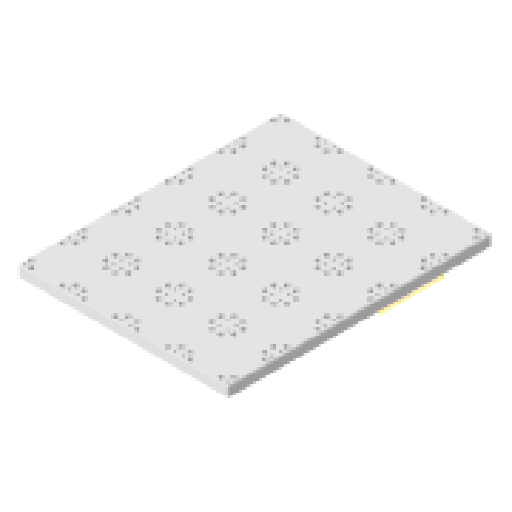
# Autodesk Inventor part: 00_Baseplate_Lightsheet
Saved by Autodesk Inventor 2025.1 (Build 291241020, 241B)
## iProperties
Created: 2024-02-01
Part Number: 00_Baseplate_Lightsheet
Material: Generisch
Document SubType Name: Modeling
Designer: diederichbenedict
Density: 1 g/cm^3
Appearance: Vorgabe
Author: diederichbenedict
Autodesk Inventor part; units mm, degrees
ref_plane "YZ Plane" through (0, 0, 0) normal (1, 0, 0) x (0, 1, 0)
ref_plane "XZ Plane" through (0, 0, 0) normal (0, 1, 0) x (-1, 0, 0)
ref_plane "XY Plane" through (0, 0, 0) normal (0, 0, 1) x (1, 0, 0)
ref_plane "Arbeitsebene1" through (0, 0, 0) normal (0, 0, 1) x (1, 0, 0)
sketch "Skizze1" plane through (0, 0, 0) normal (0, 0, 1) x (1, 0, 0)
  circle A0 centre (27, 33.3) radius 3 construction
  circle A1 centre (-8.3, 27) radius 3 construction
  circle A2 centre (-2, -8.3) radius 3 construction
  circle A3 centre (33.3, -2) radius 3 construction
  circle A4 centre (27, -8.3) radius 3 construction
  circle A5 centre (-8.3, -2) radius 3 construction
  circle A6 centre (-2, 33.3) radius 3 construction
  circle A7 centre (33.3, 27) radius 3 construction
  line L0 (27.5, 29.5) -> (-2.5, 29.5) construction
  arc A8 (29.5, 27.5) -> (27.5, 29.5) centre (27.5, 27.5) ccw construction
  line L1 (29.5, 27.5) -> (29.5, -2.5) construction
  arc A9 (27.5, -4.5) -> (29.5, -2.5) centre (27.5, -2.5) ccw construction
  line L2 (-2.5, -4.5) -> (27.5, -4.5) construction
  arc A10 (-4.5, -2.5) -> (-2.5, -4.5) centre (-2.5, -2.5) ccw construction
  line L3 (-4.5, -2.5) -> (-4.5, 27.5) construction
  arc A11 (-2.5, 29.5) -> (-4.5, 27.5) centre (-2.5, 27.5) ccw construction
  circle A12 centre (33.5, 33.5) radius 2.5 construction
  circle A13 centre (-8.5, -8.5) radius 2.5 construction
  circle A14 centre (33.5, -8.5) radius 2.5 construction
  circle A15 centre (-8.5, 33.5) radius 2.5 construction
  line L4 (-11.75, -10.5) -> (-11.75, 8.25) construction
  arc A16 (-11.75, -10.5) -> (-10.5, -11.75) centre (-10.5, -10.5) ccw construction
  line L5 (8.25, -11.75) -> (-10.5, -11.75) construction
  line L6 (8.25, -13.8774) -> (8.25, -11.75) construction
  arc A17 (7.4056, -14.8652) -> (8.25, -13.8774) centre (7.25, -13.8774) ccw construction
  arc A18 (7.4056, -14.8652) -> (7.6, -17.35) centre (7.6, -16.1) ccw construction
  line L7 (17.4, -17.35) -> (7.6, -17.35) construction
  arc A19 (17.4, -17.35) -> (17.5944, -14.8652) centre (17.4, -16.1) ccw construction
  arc A20 (16.75, -13.8774) -> (17.5944, -14.8652) centre (17.75, -13.8774) ccw construction
  line L8 (16.75, -11.75) -> (16.75, -13.8774) construction
  line L9 (35.5, -11.75) -> (16.75, -11.75) construction
  arc A21 (35.5, -11.75) -> (36.75, -10.5) centre (35.5, -10.5) ccw construction
  line L10 (36.75, 6.4875) -> (36.75, -10.5) construction
  arc A22 (36.75, 6.4875) -> (36.556, 6.5217) centre (36.65, 6.4875) ccw construction
  arc A23 (31.3, 7.45) -> (36.556, 6.5217) centre (34.01, 7.45) ccw construction
  line L11 (31.3, 17.55) -> (31.3, 7.45) construction
  arc A24 (36.556, 18.4783) -> (31.3, 17.55) centre (34.01, 17.55) ccw construction
  arc A25 (36.556, 18.4783) -> (36.75, 18.5125) centre (36.65, 18.5125) ccw construction
  line L12 (36.75, 35.5) -> (36.75, 18.5125) construction
  arc A26 (36.75, 35.5) -> (35.5, 36.75) centre (35.5, 35.5) ccw construction
  line L13 (18.5125, 36.75) -> (35.5, 36.75) construction
  arc A27 (18.5125, 36.75) -> (18.4783, 36.556) centre (18.5125, 36.65) ccw construction
  arc A28 (17.55, 31.3) -> (18.4783, 36.556) centre (17.55, 34.01) ccw construction
  line L14 (7.45, 31.3) -> (17.55, 31.3) construction
  arc A29 (6.5217, 36.556) -> (7.45, 31.3) centre (7.45, 34.01) ccw construction
  arc A30 (6.5217, 36.556) -> (6.4875, 36.75) centre (6.4875, 36.65) ccw construction
  line L15 (-10.5, 36.75) -> (6.4875, 36.75) construction
  arc A31 (-10.5, 36.75) -> (-11.75, 35.5) centre (-10.5, 35.5) ccw construction
  line L16 (-11.75, 16.75) -> (-11.75, 35.5) construction
  line L17 (-13.8774, 16.75) -> (-11.75, 16.75) construction
  arc A32 (-14.8652, 17.5944) -> (-13.8774, 16.75) centre (-13.8774, 17.75) ccw construction
  arc A33 (-14.8652, 17.5944) -> (-17.35, 17.4) centre (-16.1, 17.4) ccw construction
  line L18 (-17.35, 7.6) -> (-17.35, 17.4) construction
  arc A34 (-17.35, 7.6) -> (-14.8652, 7.4056) centre (-16.1, 7.6) ccw construction
  arc A35 (-13.8774, 8.25) -> (-14.8652, 7.4056) centre (-13.8774, 7.25) ccw construction
  line L19 (-11.75, 8.25) -> (-13.8774, 8.25) construction
  line L20 (-12.5, 7.5) -> (-12.5, -10.5) construction
  line L21 (-12.5, 7.5) -> (-12.5, -10.5)
  line L22 (-10.5, -12.5) -> (7.5, -12.5)
  line L23 (7.5, -12.5) -> (7.5, -13.8774)
  arc A36 (7.2889, -14.1243) -> (7.5, -13.8774) centre (7.25, -13.8774) ccw construction
  arc A37 (7.2889, -14.1243) -> (7.6, -18.1) centre (7.6, -16.1) ccw construction
  line L24 (7.6, -18.1) -> (17.4, -18.1) construction
  arc A38 (17.4, -18.1) -> (17.7111, -14.1243) centre (17.4, -16.1) ccw construction
  arc A39 (17.5, -13.8774) -> (17.7111, -14.1243) centre (17.75, -13.8774) ccw construction
  line L25 (17.5, -13.8774) -> (17.5, -12.5)
  line L26 (17.5, -12.5) -> (35.5, -12.5)
  line L27 (37.5, -10.5) -> (37.5, 6.4875) construction
  arc A40 (37.5, 6.4875) -> (35.8514, 6.7786) centre (36.65, 6.4875) ccw
  arc A41 (32.05, 7.45) -> (35.8514, 6.7786) centre (34.01, 7.45) ccw
  line L28 (32.05, 7.45) -> (32.05, 17.55)
  arc A42 (35.8514, 18.2214) -> (32.05, 17.55) centre (34.01, 17.55) ccw
  arc A43 (35.8514, 18.2214) -> (37.5, 18.5125) centre (36.65, 18.5125) ccw
  line L29 (37.5, 18.5125) -> (37.5, 35.5)
  line L30 (35.5, 37.5) -> (18.5125, 37.5)
  arc A44 (18.5125, 37.5) -> (18.2214, 35.8514) centre (18.5125, 36.65) ccw
  arc A45 (17.55, 32.05) -> (18.2214, 35.8514) centre (17.55, 34.01) ccw
  line L31 (17.55, 32.05) -> (7.45, 32.05)
  arc A46 (6.7786, 35.8514) -> (7.45, 32.05) centre (7.45, 34.01) ccw
  arc A47 (6.7786, 35.8514) -> (6.4875, 37.5) centre (6.4875, 36.65) ccw
  line L32 (6.4875, 37.5) -> (-10.5, 37.5)
  line L33 (-12.5, 35.5) -> (-12.5, 17.5)
  line L34 (-12.5, 17.5) -> (-13.8774, 17.5) construction
  arc A48 (-14.1243, 17.7111) -> (-13.8774, 17.5) centre (-13.8774, 17.75) ccw construction
  arc A49 (-14.1243, 17.7111) -> (-18.1, 17.4) centre (-16.1, 17.4) ccw construction
  line L35 (-18.1, 17.4) -> (-18.1, 7.6) construction
  arc A50 (-18.1, 7.6) -> (-14.1243, 7.2889) centre (-16.1, 7.6) ccw construction
  arc A51 (-13.8774, 7.5) -> (-14.1243, 7.2889) centre (-13.8774, 7.25) ccw construction
  line L36 (-13.8774, 7.5) -> (-12.5, 7.5) construction
  line L37 (-3.4722, -5.75) -> (-4.9445, -8.3) projected
  line L38 (27.5, 29.5) -> (-2.5, 29.5) projected
  arc A52 (-2.5, 29.5) -> (-4.5, 27.5) centre (-2.5, 27.5) ccw projected
  line L39 (-4.5, -2.5) -> (-4.5, 27.5) projected
  arc A53 (-4.5, -2.5) -> (-2.5, -4.5) centre (-2.5, -2.5) ccw projected
  line L40 (-2.5, -4.5) -> (27.5, -4.5) projected
  arc A54 (27.5, -4.5) -> (29.5, -2.5) centre (27.5, -2.5) ccw projected
  line L41 (29.5, 27.5) -> (29.5, -2.5) projected
  arc A55 (29.5, 27.5) -> (27.5, 29.5) centre (27.5, 27.5) ccw projected
  line L42 (33.3, 29.9445) -> (30.75, 28.4722) projected
  line L43 (30.75, 28.4722) -> (30.75, 25.5278) projected
  line L44 (30.75, 25.5278) -> (33.3, 24.0555) projected
  line L45 (33.3, 24.0555) -> (35.85, 25.5278) projected
  line L46 (35.85, 25.5278) -> (35.85, 28.4722) projected
  line L47 (35.85, 28.4722) -> (33.3, 29.9445) projected
  line L48 (24.0555, 33.3) -> (25.5278, 30.75) projected
  line L49 (25.5278, 30.75) -> (28.4722, 30.75) projected
  line L50 (28.4722, 30.75) -> (29.9445, 33.3) projected
  line L51 (29.9445, 33.3) -> (28.4722, 35.85) projected
  line L52 (28.4722, 35.85) -> (25.5278, 35.85) projected
  line L53 (25.5278, 35.85) -> (24.0555, 33.3) projected
  line L54 (33.3, -4.9445) -> (30.75, -3.4722) projected
  line L55 (35.85, -3.4722) -> (33.3, -4.9445) projected
  line L56 (35.85, -0.5278) -> (35.85, -3.4722) projected
  line L57 (33.3, 0.9445) -> (35.85, -0.5278) projected
  line L58 (30.75, -0.5278) -> (33.3, 0.9445) projected
  line L59 (30.75, -3.4722) -> (30.75, -0.5278) projected
  line L60 (24.0555, -8.3) -> (25.5278, -5.75) projected
  line L61 (25.5278, -10.85) -> (24.0555, -8.3) projected
  line L62 (28.4722, -10.85) -> (25.5278, -10.85) projected
  line L63 (29.9445, -8.3) -> (28.4722, -10.85) projected
  line L64 (28.4722, -5.75) -> (29.9445, -8.3) projected
  line L65 (25.5278, -5.75) -> (28.4722, -5.75) projected
  line L66 (-8.3, 29.9445) -> (-5.75, 28.4722) projected
  line L67 (-10.85, 28.4722) -> (-8.3, 29.9445) projected
  line L68 (-10.85, 25.5278) -> (-10.85, 28.4722) projected
  line L69 (-8.3, 24.0555) -> (-10.85, 25.5278) projected
  line L70 (-5.75, 25.5278) -> (-8.3, 24.0555) projected
  line L71 (-5.75, 28.4722) -> (-5.75, 25.5278) projected
  line L72 (0.9445, 33.3) -> (-0.5278, 30.75) projected
  line L73 (-0.5278, 35.85) -> (0.9445, 33.3) projected
  line L74 (-3.4722, 35.85) -> (-0.5278, 35.85) projected
  line L75 (-4.9445, 33.3) -> (-3.4722, 35.85) projected
  line L76 (-3.4722, 30.75) -> (-4.9445, 33.3) projected
  line L77 (-0.5278, 30.75) -> (-3.4722, 30.75) projected
  line L78 (0.9445, -8.3) -> (-0.5278, -5.75) projected
  line L79 (-0.5278, -5.75) -> (-3.4722, -5.75) projected
  line L80 (-3.4722, -5.75) -> (-4.9445, -8.3) projected
  line L81 (-4.9445, -8.3) -> (-3.4722, -10.85) projected
  line L82 (-3.4722, -10.85) -> (-0.5278, -10.85) projected
  line L83 (-0.5278, -10.85) -> (0.9445, -8.3) projected
  line L84 (-8.3, -4.9445) -> (-5.75, -3.4722) projected
  line L85 (-5.75, -3.4722) -> (-5.75, -0.5278) projected
  line L86 (-5.75, -0.5278) -> (-8.3, 0.9445) projected
  line L87 (-8.3, 0.9445) -> (-10.85, -0.5278) projected
  line L88 (-10.85, -0.5278) -> (-10.85, -3.4722) projected
  line L89 (-10.85, -3.4722) -> (-8.3, -4.9445) projected
  circle A56 centre (33.5, 33.5) radius 2.5 construction
  circle A57 centre (-8.5, -8.5) radius 2.5 construction
  circle A58 centre (33.5, -8.5) radius 2.5 construction
  circle A59 centre (-8.5, 33.5) radius 2.5 construction
  line L90 (16.75, -11.75) -> (35.5, -11.75) projected
  line L91 (16.75, -13.8774) -> (16.75, -11.75) projected
  arc A60 (16.75, -13.8774) -> (17.5944, -14.8652) centre (17.75, -13.8774) ccw construction
  arc A61 (17.4, -17.35) -> (17.5944, -14.8652) centre (17.4, -16.1) ccw construction
  line L92 (7.6, -17.35) -> (17.4, -17.35) construction
  arc A62 (7.4056, -14.8652) -> (7.6, -17.35) centre (7.6, -16.1) ccw construction
  arc A63 (7.4056, -14.8652) -> (8.25, -13.8774) centre (7.25, -13.8774) ccw construction
  line L93 (8.25, -11.75) -> (8.25, -13.8774) projected
  line L94 (-10.5, -11.75) -> (8.25, -11.75) projected
  arc A64 (-11.75, -10.5) -> (-10.5, -11.75) centre (-10.5, -10.5) ccw projected
  line L95 (-11.75, 8.25) -> (-11.75, -10.5) projected
  line L96 (-13.8774, 8.25) -> (-11.75, 8.25) construction
  arc A65 (-13.8774, 8.25) -> (-14.8652, 7.4056) centre (-13.8774, 7.25) ccw construction
  arc A66 (-17.35, 7.6) -> (-14.8652, 7.4056) centre (-16.1, 7.6) ccw construction
  line L97 (-17.35, 17.4) -> (-17.35, 7.6) construction
  arc A67 (-14.8652, 17.5944) -> (-17.35, 17.4) centre (-16.1, 17.4) ccw construction
  arc A68 (-14.8652, 17.5944) -> (-13.8774, 16.75) centre (-13.8774, 17.75) ccw construction
  line L98 (-11.75, 16.75) -> (-13.8774, 16.75) construction
  line L99 (-11.75, 35.5) -> (-11.75, 16.75) projected
  arc A69 (-10.5, 36.75) -> (-11.75, 35.5) centre (-10.5, 35.5) ccw projected
  line L100 (6.4875, 36.75) -> (-10.5, 36.75) projected
  arc A70 (6.5217, 36.556) -> (6.4875, 36.75) centre (6.4875, 36.65) ccw projected
  arc A71 (6.5217, 36.556) -> (7.45, 31.3) centre (7.45, 34.01) ccw projected
  line L101 (17.55, 31.3) -> (7.45, 31.3) projected
  arc A72 (17.55, 31.3) -> (18.4783, 36.556) centre (17.55, 34.01) ccw projected
  arc A73 (18.5125, 36.75) -> (18.4783, 36.556) centre (18.5125, 36.65) ccw projected
  line L102 (35.5, 36.75) -> (18.5125, 36.75) projected
  arc A74 (36.75, 35.5) -> (35.5, 36.75) centre (35.5, 35.5) ccw projected
  line L103 (36.75, 18.5125) -> (36.75, 35.5) projected
  arc A75 (36.556, 18.4783) -> (36.75, 18.5125) centre (36.65, 18.5125) ccw projected
  arc A76 (36.556, 18.4783) -> (31.3, 17.55) centre (34.01, 17.55) ccw projected
  line L104 (31.3, 7.45) -> (31.3, 17.55) projected
  arc A77 (31.3, 7.45) -> (36.556, 6.5217) centre (34.01, 7.45) ccw projected
  arc A78 (36.75, 6.4875) -> (36.556, 6.5217) centre (36.65, 6.4875) ccw projected
  line L105 (36.75, -10.5) -> (36.75, 6.4875) projected
  arc A79 (35.5, -11.75) -> (36.75, -10.5) centre (35.5, -10.5) ccw projected
  line L106 (33.5, -8.5) -> (33.5, 33.5) construction
  line L107 (33.5, 33.5) -> (-8.5, 33.5) construction
  line L108 (-8.5, 33.5) -> (-8.5, -8.5) construction
  circle A80 centre (-8.5, -8.5) radius 1.4
  circle A81 centre (-8.5, 33.5) radius 1.4
  circle A82 centre (33.5, 33.5) radius 1.4
  circle A83 centre (33.5, -8.5) radius 1.4
  line L109 (37.5, -10.5) -> (37.5, -12.5)
  line L110 (37.5, -12.5) -> (35.4967, -12.5)
  line L111 (-10.5, -12.5) -> (-12.5, -12.5)
  line L112 (-12.5, -12.5) -> (-12.5, -10.5)
  line L113 (-12.5, 35.5) -> (-12.5, 37.5)
  line L114 (-12.5, 37.5) -> (-10.5, 37.5)
  line L115 (37.5, 35.5) -> (37.5, 37.5)
  line L116 (37.5, 37.5) -> (35.5, 37.5)
  circle A84 centre (12.5, 12.5) radius 25 construction
  line L117 (-8.5, 33.5) -> (33.5, 33.5) construction
  line L118 (33.5, 33.5) -> (33.5, -8.5) construction
  line L119 (33.5, -8.5) -> (-8.5, -8.5) construction
  line L120 (-8.5, -8.5) -> (-8.5, 33.5) construction
  line L121 (-8.5, 33.5) -> (33.5, -8.5) construction
  line L122 (33.5, 33.5) -> (-8.5, -8.5) construction
  line L123 (37.5, -10.5) -> (37.5, 18.5125)
  arc A85 (18.5125, -12.5) -> (18.2214, -14.1486) centre (18.5125, -13.35) ccw
  arc A86 (17.55, -17.95) -> (18.2214, -14.1486) centre (17.55, -15.99) ccw construction
  line L124 (17.55, -17.95) -> (7.45, -17.95) construction
  arc A87 (6.7786, -14.1486) -> (7.45, -17.95) centre (7.45, -15.99) ccw construction
  arc A88 (6.7786, -14.1486) -> (6.4875, -12.5) centre (6.4875, -13.35) ccw
  line L125 (37.5, 37.5) -> (-12.5, 37.5)
  line L126 (-12.5, 37.5) -> (-12.5, -12.5)
  line L127 (-12.5, -12.5) -> (37.5, -12.5)
  line L128 (37.5, -12.5) -> (37.5, 37.5)
  point P0 (0, 0)
  point P1 (6.4875, -12.5)
  point P2 (6.0394, -17.3508)
  point P3 (18.9606, -17.3508)
  point P4 (18.5125, -12.5)
  point P5 (37.5, 6.4875)
  point P6 (18.5125, 37.5)
  point P7 (6.4875, 37.5)
  point P8 (-12.5, 17.5)
  point P9 (-10.4995, -12.5)
  dimension "d17" = 2.8
  dimension "d18" = 2.8
  dimension "d19" = 2.8
  dimension "d20" = 2.8
  dimension "d53" = 42
  dimension "d54" = 42
  constraints: 78 end point, 40 point on circle, 25 centre point, 5 collinear, 5 parallel, 4 coincident, 4 perpendicular, 3 horizontal, 3 tangent, 2 midpoint, 1 point on line, 1 vertical, 27 other
  measures "d17" diameter of A80
  measures "d18" diameter of A81
  measures "d19" diameter of A82
  measures "d20" diameter of A83
  measures "d53" distance of L106.start L119.end
  measures "d54" distance of L117.end L106.start
extrude "Extrusion1" add sketch "Skizze1" along normal blind 10.5 contours L126 L33 L113 L114 L32 A47 A46 L31 A45 A44 L30 L116 L115 L29 A43 A42 L28 A41 A40 L123 L109 L110 L26 L127 L22 L111 L112 L21 | L125 A44 A45 L31 A46 A47 | L123 A40 A41 L28 A42 A43 | A55 L41 A54 L40 A53 L39 A52 L38
sketch "Skizze3" plane through (0, 0, 10.5) normal (0, 0, 1) x (1, 0, 0)
  circle A0 centre (33.5, -8.5) radius 1.4 projected
  circle A1 centre (-8.5, -8.5) radius 1.4 projected
  circle A2 centre (-8.5, 33.5) radius 1.4 projected
  circle A3 centre (33.5, 33.5) radius 1.4 projected
  point P0 (0, 0)
hole "Bohrung1" at (33.5, -8.5, 10.5) at (-8.5, -8.5, 10.5) at (-8.5, 33.5, 10.5) at (33.5, 33.5, 10.5) direction (0, 0, -1) diameter 3.3 end through all
pattern_linear "Rechteckige Anordnung4" count 4 spacing 50 along (-1, 0, 0) count 4 spacing 50 along (0, -1, 0) of "Extrusion1", "Bohrung1"
pattern_linear "Rechteckige Anordnung7" count 2 spacing 50 along (0, 1, 0) count 4 spacing 50 along (-1, 0, 0) of "Extrusion1"
chamfer "Chamfer1" distance 1 angle 45 38 edges at (-62.5, -162.5, 10.5) (37.5, -37.5, 10.5) (-62.5, 87.5, 10.5) (-162.5, -161.5, 10.5) (-162.5, -151.5, 10.5) (-162.5, -137.5, 10.5) (-162.5, -121.5, 10.5) (-162.5, -101.5, 10.5) (-162.5, -87.5, 10.5) (-162.5, -71.5, 10.5) (-162.5, -51.5, 10.5) (-162.5, -37.5, 10.5) (-162.5, -21.5, 10.5) (-162.5, 77.5, 10.5) (-162.5, 62.5, 10.5) (-162.5, 48.5, 10.5) (-162.5, 28.5, 10.5) (-162.5, 12.5, 10.5) (-162.5, -1.5, 10.5) (-62.5, 87.5, 0) (-162.5, 77.5, 0) (-162.5, 62.5, 0) (-162.5, 48.5, 0) (-162.5, 28.5, 0) (-162.5, 12.5, 0) (-162.5, -1.5, 0) (-162.5, -21.5, 0) (-162.5, -37.5, 0) (-162.5, -51.5, 0) (-162.5, -71.5, 0) (-162.5, -87.5, 0) (-162.5, -101.5, 0) (-162.5, -121.5, 0) (-162.5, -137.5, 0) (-162.5, -151.5, 0) (-162.5, -161.5, 0) (37.5, -37.5, 0) (-62.5, -162.5, 0)
fillet "Fillet3" radius 3 4 edges at (-162.5, 87.5, 5.25) (37.5, 87.5, 5.25) (-162.5, -162.5, 5.25) (37.5, -162.5, 5.25)
